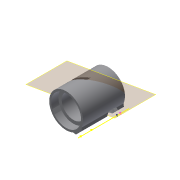
# Autodesk Inventor part: 30_focus_inlet_objective_mount_v7
Saved by Autodesk Inventor 2019 (Build 230136000, 136)
## iProperties
Created: 2019-10-25
Part Number: 30_focus_inlet_objective_mount_v7
Material: Generic
Document SubType Name: Modeling
Designer: marsikovabarbora
Density: 1 g/cm^3
Appearance: Default
Mass: 5.76385 g
Surface Area: 46.4248 cm^2
Volume: 5.76385 cm^3
Author: marsikovabarbora
Autodesk Inventor part; units mm, degrees
ref_plane "YZ Plane" through (0, 0, 0) normal (1, 0, 0) x (0, 1, 0)
ref_plane "XZ Plane" through (0, 0, 0) normal (0, 1, 0) x (-1, 0, 0)
sketch "Sketch1" plane through (0, 0, 0) normal (0, 0, 1) x (1, 0, 0)
  line L0 (9.680091, -14.007986) -> (7.205218, -11.533112) construction
  line L1 (7.205218, -11.533112) -> (11.58928, -7.14905) construction
  line L2 (11.58928, -7.14905) -> (14.064153, -9.623924) construction
  line L3 (14.064153, -9.623924) -> (9.680091, -14.007986) construction
  arc A0 (12.636919, -4.749554) -> (4.749554, -12.636919) centre (0, 0) ccw construction
  line L4 (10.929756, -3.042391) -> (12.636919, -4.749554) construction
  line L5 (11.661769, -4.612198) -> (10.929756, -3.042391) construction
  arc A1 (11.661769, -4.612198) -> (10.855062, -4.469954) centre (11.208615, -4.823507) ccw construction
  line L6 (10.791549, -4.533466) -> (10.855062, -4.469954) construction
  arc A2 (10.791549, -4.533466) -> (10.652699, -4.973844) centre (11.145103, -4.88702) ccw construction
  line L7 (10.914957, -6.461185) -> (10.652699, -4.973844) construction
  arc A3 (10.776107, -6.901563) -> (10.914957, -6.461185) centre (10.422553, -6.548009) ccw construction
  line L8 (6.901563, -10.776107) -> (10.776107, -6.901563) construction
  arc A4 (6.461185, -10.914957) -> (6.901563, -10.776107) centre (6.548009, -10.422553) ccw construction
  line L9 (6.461185, -10.914957) -> (4.973844, -10.652699) construction
  arc A5 (4.973844, -10.652699) -> (4.533466, -10.791549) centre (4.88702, -11.145103) ccw construction
  line L10 (4.533466, -10.791549) -> (4.469954, -10.855062) construction
  arc A6 (4.469954, -10.855062) -> (4.612198, -11.661769) centre (4.823507, -11.208615) ccw construction
  line L11 (4.612198, -11.661769) -> (3.042391, -10.929756) construction
  line L12 (3.042391, -10.929756) -> (4.749554, -12.636919) construction
  line L13 (-1.716744, -14.649754) -> (-1.716744, -17.5) construction
  line L14 (-1.716744, -17.5) -> (1.716744, -17.5) construction
  line L15 (1.716744, -14.649754) -> (1.716744, -17.5) construction
  arc A7 (1.716744, -14.649754) -> (6.959526, -13.004903) centre (0, 0) ccw construction
  arc A8 (6.959526, -13.004903) -> (8.272803, -15.178914) centre (8.299448, -13.679151) ccw construction
  line L16 (8.272803, -15.178914) -> (7.681619, -15.168411) construction
  arc A9 (8.524943, -17.890121) -> (7.681619, -15.168411) centre (7.654974, -16.668175) ccw construction
  line L17 (8.524943, -17.890121) -> (13.516139, -14.336623) construction
  line L18 (13.516139, -14.336623) -> (13.516139, -12.282269) construction
  line L19 (13.516139, -12.282269) -> (14.616822, -12.282269) construction
  line L20 (14.616822, -12.282269) -> (14.616822, -1.977626) construction
  arc A10 (14.616822, -1.977626) -> (1.716744, 14.649754) centre (0, 0) ccw construction
  line L21 (1.716744, 14.649754) -> (1.716744, 17.5) construction
  line L22 (-1.716744, 17.5) -> (1.716744, 17.5) construction
  line L23 (-1.716744, 14.649754) -> (-1.716744, 17.5) construction
  arc A11 (-1.716744, 14.649754) -> (-14.281691, -3.68725) centre (0, 0) ccw construction
  line L24 (-14.281691, -3.68725) -> (-15.413484, -5.793543) construction
  arc A12 (-15.413484, -5.793543) -> (-14.598383, -8.501976) centre (-13.651717, -6.740209) ccw construction
  line L25 (-14.598383, -8.501976) -> (-9.632638, -11.170264) construction
  arc A13 (-9.632638, -11.170264) -> (-1.716744, -14.649754) centre (0, 0) ccw construction
  line L26 (-24.6, 24.6) -> (25.2, -25.2) construction
  line L27 (25.2, 24.6) -> (-24.6, -25.2) construction
  arc A14 (-1.428286, 10.15) -> (-9.504301, -3.838068) centre (0, 0) ccw
  circle A15 centre (0, 0) radius 10.1 construction
  line L28 (-1.428286, 10.15) -> (1.428286, 10.15)
  line L29 (-8.076015, -6.311932) -> (-9.504301, -3.838068)
  line L30 (9.504301, -3.838068) -> (8.076015, -6.311932)
  arc A16 (1.428286, 10.15) -> (-1.428286, 10.15) centre (0, 0) ccw
  arc A17 (9.504301, -3.838068) -> (1.428286, 10.15) centre (0, 0) ccw
  arc A18 (8.076015, -6.311932) -> (9.504301, -3.838068) centre (0, 0) ccw
  arc A19 (-8.076015, -6.311932) -> (8.076015, -6.311932) centre (0, 0) ccw
  arc A20 (-9.504301, -3.838068) -> (-8.076015, -6.311932) centre (0, 0) ccw
  arc A21 (10.705396, -6.830852) -> (10.816477, -6.47855) centre (10.422553, -6.548009) ccw
  line L31 (10.816477, -6.47855) -> (10.554218, -4.991208)
  arc A22 (10.720839, -4.462755) -> (10.595608, -4.646072) centre (11.145103, -4.88702) ccw construction
  line L32 (10.720839, -4.462755) -> (10.784351, -4.399243) construction
  arc A23 (11.760139, -5.059773) -> (10.784351, -4.399243) centre (11.208615, -4.823507) ccw construction
  line L33 (11.760139, -5.059773) -> (10.599447, -2.57066) construction
  line L34 (10.599447, -2.57066) -> (12.597204, -4.568418) construction
  arc A24 (12.597204, -4.568418) -> (4.568418, -12.597204) centre (0, 0) ccw construction
  line L35 (4.568418, -12.597204) -> (2.57066, -10.599447) construction
  line L36 (2.57066, -10.599447) -> (4.249147, -11.382138) construction
  arc A25 (4.399243, -10.784351) -> (4.249147, -11.382138) centre (4.823507, -11.208615) ccw construction
  line L37 (4.399243, -10.784351) -> (4.462755, -10.720839) construction
  arc A26 (4.991208, -10.554218) -> (4.646072, -10.595608) centre (4.88702, -11.145103) ccw
  line L38 (4.991208, -10.554218) -> (6.47855, -10.816477)
  arc A27 (6.47855, -10.816477) -> (6.830852, -10.705396) centre (6.548009, -10.422553) ccw
  line L39 (6.830852, -10.705396) -> (10.705396, -6.830852)
  circle A28 centre (0, 0) radius 11.569481
  arc A29 (4.646072, -10.595608) -> (4.462755, -10.720839) centre (4.88702, -11.145103) ccw construction
  arc A30 (10.595608, -4.646072) -> (10.554218, -4.991208) centre (11.145103, -4.88702) ccw
  dimension "d4" = 20.2
  dimension "d5" = 10.15
  dimension "d6" = 20.5
  dimension "d9" = 360
  dimension "d11" = 0.1
  constraints: 32 point on circle, 24 end point, 17 centre point, 4 tangent, 3 coincident, 1 horizontal, 21 other
  measures "d4" diameter of A15
  measures "d5" distance from line of L28 point (0, 0)
  measures "d6" diameter of A14
  measures "d11" distance between parallel lines of L8 L39
extrude "Extrusion1" add sketch "Sketch1" against normal blind 5 contours A16 L28 | L29 A20 | A18 L30 | L39 A27 L38 A26 A28 A30 L31 A21 | A28
sketch "Sketch3" plane through (0, 0, -5) normal (0, 0, -1) x (-1, 0, 0)
  line L0 (9.504301, -3.838068) -> (8.076015, -6.311932)
  arc A0 (-8.076015, -6.311932) -> (8.076015, -6.311932) centre (0, 0) ccw
  line L1 (-8.076015, -6.311932) -> (-9.504301, -3.838068)
  arc A1 (-1.428286, 10.15) -> (-9.504301, -3.838068) centre (0, 0) ccw
  line L2 (-1.428286, 10.15) -> (1.428286, 10.15)
  arc A2 (9.504301, -3.838068) -> (1.428286, 10.15) centre (0, 0) ccw
  arc A3 (-10.816477, -6.47855) -> (-10.705396, -6.830852) centre (-10.422553, -6.548009) ccw
  line L3 (-10.705396, -6.830852) -> (-6.830852, -10.705396)
  arc A4 (-6.830852, -10.705396) -> (-6.47855, -10.816477) centre (-6.548009, -10.422553) ccw
  line L4 (-6.47855, -10.816477) -> (-4.991208, -10.554218)
  arc A5 (-4.646072, -10.595608) -> (-4.991208, -10.554218) centre (-4.88702, -11.145103) ccw
  arc A6 (-4.646072, -10.595608) -> (-10.595608, -4.646072) centre (0, 0) ccw
  arc A7 (-10.554218, -4.991208) -> (-10.595608, -4.646072) centre (-11.145103, -4.88702) ccw
  line L5 (-10.554218, -4.991208) -> (-10.816477, -6.47855)
  circle A8 centre (0, 0) radius 8
  circle A9 centre (0, 0) radius 10.25
  dimension "d17" = 16
  constraints: 2 centre point, 2 coincident, 1 concentric
  measures "d17" diameter of A8
extrude "Extrusion3" add sketch "Sketch3" along normal blind 4 contours A9 L0 | L0 A0 L1 A1 L2 A2 | A9 L1 | L2 A9 | L5 A7 A6 A5 L4 A4 L3 A3
sketch "Sketch4" plane through (6.830852, -10.705396, 0) normal (0.7071068, -0.7071068, 0) x (0, 0, -1)
  line L0 (0, 0) -> (0, 5.479433) construction
  line L1 (0, 0) -> (9, 0) construction
  line L2 (9, 5.479433) -> (9, 0) construction
  line L3 (0, 5.479433) -> (9, 5.479433) construction
  line L4 (0, 2.739716) -> (9, 2.739716) construction
  circle A0 centre (7.2, 2.739716) radius 1.4
  dimension "d20" = 2.8
  dimension "d21" = 1.8
  constraints: 2 end point, 1 centre point, 1 midpoint, 1 point on line
  measures "d20" diameter of A0
  measures "d21" distance from line of L2 A0.centre
extrude "Extrusion4" cut sketch "Sketch4" against normal up to surface round surface about axis through (0, 0, -5) along (0, 0, -1) radius 8 far side no
sketch "Sketch5" plane through (0, 0, -9) normal (0, 0, -1) x (-1, 0, 0)
  circle A0 centre (0, 0) radius 8
  arc A1 (-10.816477, -6.47855) -> (-10.705396, -6.830852) centre (-10.422553, -6.548009) ccw
  line L0 (-10.705396, -6.830852) -> (-6.830852, -10.705396)
  arc A2 (-6.830852, -10.705396) -> (-6.47855, -10.816477) centre (-6.548009, -10.422553) ccw
  line L1 (-6.47855, -10.816477) -> (-4.991208, -10.554218)
  arc A3 (-4.646072, -10.595608) -> (-4.991208, -10.554218) centre (-4.88702, -11.145103) ccw
  arc A4 (-4.646072, -10.595608) -> (-10.595608, -4.646072) centre (0, 0) ccw
  arc A5 (-10.554218, -4.991208) -> (-10.595608, -4.646072) centre (-11.145103, -4.88702) ccw
  line L2 (-10.554218, -4.991208) -> (-10.816477, -6.47855)
extrude "Extrusion5" add sketch "Sketch5" along normal up to surface (19.779423 mm away)
ref_plane "Work Plane1" through (0.364322, -11.678031, -30.384776) normal (0.5, -0.5, 0.7071068) x (-0.7071068, -0.7071068, 0)
sketch "Sketch6" plane through (0.364322, -11.678031, -30.384776) normal (0.5, -0.5, 0.7071068) x (-0.7071068, -0.7071068, 0)
  line L0 (-16, 0) -> (0, 0)
  line L1 (0, 0) -> (0, -25)
  line L2 (-16, -25) -> (-16, 0)
  line L3 (0, -25) -> (-16, -25)
  line L4 (0.5, 0.5) -> (-16.5, 0.5)
  line L5 (-16.5, 0.5) -> (-16.5, -25.5)
  line L6 (-16.5, -25.5) -> (0.5, -25.5)
  line L7 (0.5, -25.5) -> (0.5, 0.5)
  line L8 (0.5, 0.5) -> (-16.5, 0.5)
  line L9 (-16.5, 0.5) -> (-16.5, 6.511713)
  line L10 (-16.5, 6.511713) -> (0.5, 6.511713)
  line L11 (0.5, 6.511713) -> (0.5, 0.5)
  line L12 (0.5, -25.5) -> (-16.5, -25.5)
  line L13 (-16.5, -25.5) -> (-16.5, -35.466293)
  line L14 (-16.5, -35.466293) -> (0.5, -35.466293)
  line L15 (0.5, -35.466293) -> (0.5, -25.5)
  point P0 (-8, -27.506458)
  dimension "d38" = 0.5
  constraints: 32 end point, 4 horizontal, 4 parallel, 2 perpendicular, 2 vertical, 7 other
  measures "d38" distance between parallel lines of L0 L4
extrude "Extrusion6" cut sketch "Sketch6" against normal blind 1.7 contours L0 L1 L3 L2 | L7 L6 L5 L4 | L4 L9 L10 L11 | L15 L14 L13 L6
sketch "Sketch7" plane through (6.830852, -10.705396, 0) normal (0.7071068, -0.7071068, 0) x (-0.7071068, -0.7071068, 0)
  arc A0 (-1.614475, 20.869748) -> (-3.864958, 20.869748) centre (-2.739716, 21.192388) ccw
  circle A1 centre (-2.739716, 21.192388) radius 4.5
  point P0 (-2.739716, 0)
  dimension "d39" = 9
  constraints: 2 centre point, 2 point on circle, 1 coincident, 4 other
  measures "d39" diameter of A1
extrude "Extrusion7" cut sketch "Sketch7" against normal blind 10
sketch "Sketch8" plane through (10.705396, -6.830852, 0) normal (0.7071068, -0.7071068, 0) x (-0.7071068, -0.7071068, 0)
  line L0 (10.739716, 28.779423) -> (-5.260284, 28.779423)
  line L1 (-2.760284, 9.605354) -> (8.239716, 9.605354)
  line L2 (8.239716, 9.605354) -> (8.239716, 28.779423)
  line L3 (8.239716, 28.779423) -> (-2.760284, 28.779423)
  line L4 (-2.760284, 28.779423) -> (-2.760284, 9.605354)
  line L5 (-2.760284, 9.605354) -> (8.239716, 28.779423) construction
  line L6 (8.239716, 9.605354) -> (-2.760284, 28.779423) construction
  circle A0 centre (2.739716, 21.192388) radius 2
  circle A1 centre (2.739716, 21.192388) radius 3.001655
  point P0 (2.739716, 0)
  dimension "d32" = 11
  constraints: 12 end point, 2 centre point, 2 parallel, 1 coincident, 1 horizontal, 1 perpendicular, 1 point on line, 2 other
  measures "d32" distance of L3.end L2.end
extrude "Extrusion8" add sketch "Sketch8" against normal up to surface contours L2 L1 L4 L0 round surface about axis through (0, 0, 0) along (0, 0, -1) radius 11.569481 far side no
sketch "Sketch9" plane through (12.657211, -4.879037, -9.605354) normal (0.7071068, -0.7071068, 0) x (-0.7071068, -0.7071068, 0)
  line L0 (11, 19.174069) -> (0, 19.174069)
  line L1 (2.760284, -9.605354) -> (2.760284, 0)
  line L2 (8.239716, -9.605354) -> (2.760284, -9.605354)
  line L3 (8.239716, -9.605354) -> (8.239716, 0)
  circle A0 centre (5.5, -2.405354) radius 1.4
  line L4 (0, 19.174069) -> (0, 0)
  line L5 (0, 0) -> (2.760284, 0)
  line L6 (8.239716, 0) -> (11, 0)
  line L7 (11, 0) -> (11, 19.174069)
  circle A1 centre (5.5, 11.587035) radius 2.75
  circle A2 centre (5.5, 11.587035) radius 4.75
  point P0 (5.5, -9.605354)
  dimension "d40" = 9.5
  constraints: 2 centre point, 1 coincident, 2 other
  measures "d40" diameter of A2
ref_plane "Work Plane2" through (2.218603, -17.951387, -31.242029) normal (-0.7071068, 0.7071068, 0) x (-0.3650227, -0.3650227, 0.856456)
extrude "Extrusion9" add sketch "Sketch9" along normal up to surface (1.862336 mm away) contours L7 L6 L3 L2 L1 L5 L4 L0
sketch "Sketch10" plane through (6.195907, -13.974082, -9.605354) normal (0.7071068, -0.7071068, 0) x (-0.7071068, -0.7071068, 0)
  line L0 (-8.239716, 0) -> (-8.239716, -9.605354)
  line L1 (-8.239716, -9.605354) -> (-2.760284, -9.605354)
  circle A0 centre (-5.5, -2.405354) radius 1.4
  arc A1 (-3.111277, 19.174069) -> (-1.722597, 16.423875) centre (-0.400217, 18.817293) ccw construction
  line L2 (-11, 0) -> (-8.239716, 0)
  line L3 (-2.760284, -9.605354) -> (-2.760284, 0)
  line L4 (-2.760284, 0) -> (0, 0)
  line L5 (0, 0) -> (0, 19.174069)
  line L6 (0, 19.174069) -> (-11, 19.174069)
  line L7 (-11, 19.174069) -> (-11, 0)
  point P0 (-5.5, -9.605354)
  constraints: 2 point on circle, 1 centre point, 4 other
sketch "Sketch11" plane through (10.816477, -6.47855, -9.605354) normal (0, 0, 1) x (0.9848078, 0.1736482, 0)
  arc A0 (-5.025297, -3.518751) -> (-4.659058, -3.470534) centre (-4.888489, -3.142874) ccw
  line L0 (-6.444502, -3.002202) -> (-5.025297, -3.518751)
  arc A1 (-6.444502, -3.002202) -> (-6.791582, -2.983031) centre (-6.649714, -3.566018) ccw
  arc A2 (-8.194321, -3.234063) -> (-6.791582, -2.983031) centre (-9.527162, 8.258388) ccw
  line L1 (-8.194321, -3.234063) -> (-5.851958, -6.579305)
  line L2 (-3.590866, -4.996071) -> (-5.851958, -6.579305)
  line L3 (-4.659058, -3.470534) -> (-3.590866, -4.996071)
  arc A3 (-0.170569, -0.327661) -> (0, 0) centre (-0.4, 0) ccw
  line L4 (-0.170569, -0.327661) -> (0.897623, -1.853197)
  line L5 (3.158715, -0.269964) -> (0.897623, -1.853197)
  line L6 (3.158715, -0.269964) -> (0.816352, 3.075277)
  arc A4 (0.100694, 1.842992) -> (0.816352, 3.075277) centre (-9.527162, 8.258388) ccw
  arc A5 (0.100694, 1.842992) -> (0, 1.510286) centre (0.6, 1.510286) ccw
  line L7 (0, 0) -> (0, 1.510286)
extrude "Extrusion10" cut sketch "Sketch11" against normal blind 5
sketch "Sketch12" plane through (0, 0, -28.779423) normal (0, 0, -1) x (-0.7071068, 0.7071068, 0)
  arc A0 (-10.777495, -4.206958) -> (-10.777495, 4.206958) centre (0, 0) ccw
  line L0 (-10.992277, 3.933642) -> (-12.229431, 3.067377)
  line L1 (-12.4, 2.739716) -> (-12.4, -2.739716)
  line L2 (-12.229431, -3.067377) -> (-10.992277, -3.933642)
  arc A1 (-10.992277, 3.933642) -> (-10.777495, 4.206958) centre (-11.336422, 4.425133) ccw
  arc A2 (-12.229431, 3.067377) -> (-12.4, 2.739716) centre (-12, 2.739716) ccw
  arc A3 (-12.4, -2.739716) -> (-12.229431, -3.067377) centre (-12, -2.739716) ccw
  arc A4 (-10.777495, -4.206958) -> (-10.992277, -3.933642) centre (-11.336422, -4.425133) ccw
  line L3 (-10.178551, -5.5) -> (-14.262336, -5.5)
  line L4 (-14.262336, -5.5) -> (-14.262336, 5.5)
  line L5 (-10.178551, 5.5) -> (-14.262336, 5.5)
  point P0 (0, 0)
  constraints: 10 point on circle, 6 end point, 5 centre point, 1 vertical, 20 other
extrude "Extrusion11" cut sketch "Sketch12" against normal through all contours A0 L3 L4 L5 A1 L0 A2 L1 A3 L2 A4
sketch "Sketch13" plane through (10.705396, -6.830852, 0) normal (0.7071068, -0.7071068, 0) x (-0.7071068, -0.7071068, 0)
  circle A0 centre (2.739716, 21.192388) radius 2.75
  circle A1 centre (2.739716, 21.192388) radius 4.83833
  line L0 (1.224642, 29.401251) -> (4.254791, 29.401251)
  line L1 (4.254791, 29.401251) -> (4.254791, 12.983525)
  line L2 (4.254791, 12.983525) -> (1.224642, 12.983525)
  line L3 (1.224642, 12.983525) -> (1.224642, 29.401251)
  line L4 (1.224642, 29.401251) -> (4.254791, 12.983525) construction
  line L5 (4.254791, 29.401251) -> (1.224642, 12.983525) construction
  point P0 (2.739716, 0)
  constraints: 12 end point, 2 centre point, 2 midpoint, 2 parallel, 1 coincident, 1 horizontal, 1 perpendicular, 2 other
extrude "Extrusion12" cut sketch "Sketch13" against normal blind 2
body "Solid1"
